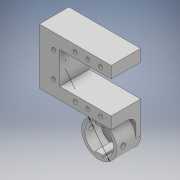
# Autodesk Inventor part: bottom
Saved by Autodesk Inventor 2018 (Build 220112000, 112)
## iProperties
Created: 2018-02-07
Part Number: bottom
Material: Générique
Document SubType Name: Modeling
Designer: Mephiro
Density: 1 g/cm^3
Appearance: Par défaut
Author: Mephiro
Autodesk Inventor part; units mm, degrees
ref_plane "YZ Plane" through (0, 0, 0) normal (1, 0, 0) x (0, 1, 0)
ref_plane "XZ Plane" through (0, 0, 0) normal (0, 1, 0) x (-1, 0, 0)
ref_plane "XY Plane" through (0, 0, 0) normal (0, 0, 1) x (1, 0, 0)
sketch "Esquisse1" plane through (0, 0, 0) normal (0, 1, 0) x (-1, 0, 0)
  circle A0 centre (0, 0) radius 11
  circle A1 centre (0, 0) radius 9.5
  dimension "d0" = 22
  dimension "d1" = 19
  constraints: 2 centre point, 2 coincident
  measures "d0" diameter of A0
  measures "d1" diameter of A1
extrude "Extrusion1" add sketch "Esquisse1" along normal blind 5 contours A0 | A1
sketch "Esquisse2" plane through (0, 0, 0) normal (0, -1, 0) x (1, 0, 0)
  circle A0 centre (0, 0) radius 11
  dimension "d5" = 22
  constraints: 1 centre point, 1 coincident
  measures "d5" diameter of A0
extrude "Extrusion2" add sketch "Esquisse2" along normal blind 10
sketch "Esquisse3" plane through (0, -10, 0) normal (0, -1, 0) x (1, 0, 0)
  arc A0 (2.4, -8.6741) -> (2.4, 8.6741) centre (0, 0) ccw
  arc A1 (-2.4, 8.6741) -> (-2.4, -8.6741) centre (0, 0) ccw
  line L0 (-2.4, -8.6741) -> (-2.4, -7.4241)
  line L1 (-2.4, -7.4241) -> (2.4, -7.4241)
  line L2 (2.4, -7.4241) -> (2.4, -8.6741)
  line L3 (-2.4, 8.6741) -> (-2.4, 7.4241)
  line L4 (-2.4, 7.4241) -> (2.4, 7.4241)
  line L5 (2.4, 7.4241) -> (2.4, 8.6741)
  dimension "d23" = 9
  dimension "d24" = 9
  dimension "d30" = 1.25
  dimension "d31" = 1.25
  dimension "d32" = 4.8
  dimension "d33" = 2.4
  dimension "d34" = 2.4
  dimension "d35" = 4.8
  constraints: 12 end point, 4 point on circle, 2 centre point, 2 parallel, 1 coincident
  measures "d23" radius of A0
  measures "d24" radius of A1
  measures "d30" distance of L1.end L2.end
  measures "d31" distance of L3.start L3.end
  measures "d32" distance of L2.end L0.start
  measures "d33" horizontal distance of L0.start point (0, 0)
  measures "d34" horizontal distance of point (0, 0) L3.start
  measures "d35" distance of L5.end L3.start
extrude "Extrusion3" cut sketch "Esquisse3" against normal blind 10
sketch "Esquisse5" plane through (0, 0, 0) normal (1, 0, 0) x (0, 1, 0)
  circle A0 centre (-6, 0) radius 1.5
  line L0 (0, -8.6741) -> (0, 8.6741) projected
  point P0 (0, 0)
  point P1 (0, -8.5184)
  point P2 (0, 8.5184)
  dimension "d26" = 3
  dimension "d27" = 6
  constraints: 1 centre point
  measures "d26" diameter of A0
  measures "d27" distance from line of L0 A0.centre
extrude "Extrusion5" cut sketch "Esquisse5" along normal mid plane 30
sketch "Esquisse14" plane through (41.6905, 5, 9.6899) normal (0, 1, 0) x (0, 0, -1)
  line L0 (-37.8101, 30.6905) -> (-2.8101, 30.6905)
  line L1 (-2.8101, 30.6905) -> (-2.8101, 75.6905)
  line L2 (-2.8101, 75.6905) -> (-37.8101, 75.6905)
  line L3 (-37.8101, 75.6905) -> (-37.8101, 30.6905)
  line L4 (-37.8101, 30.6905) -> (-37.8101, 75.6905)
  line L5 (-45, 30.6905) -> (-37.8101, 30.6905)
  circle A0 centre (9.6899, 41.6905) radius 11 projected
  point P0 (0, 0)
  dimension "d107" = 35
  dimension "d106" = 45
  dimension "d139" = 11
  dimension "d140" = 12.5
  constraints: 12 end point, 2 collinear, 2 parallel, 1 horizontal, 1 perpendicular
  measures "d107" distance of L0.start L0.end
  measures "d106" distance of L2.end L0.start
  measures "d139" distance from line of A0.centre L0
  measures "d140" distance from line of L1 A0.centre
extrude "Extrusion11" add sketch "Esquisse14" against normal blind 3 contours L3 L2 L1 L0
sketch "Esquisse18" plane through (0, 5, 12.5) normal (0, 0, -1) x (-1, 0, 0)
  line L0 (34, -3) -> (-11, -3) projected
  line L1 (11.3351, 0) -> (-11, 0)
  line L2 (-11, 0) -> (-11, -3)
  line L3 (-11, -3) -> (11.3351, -3)
  line L4 (11.3351, -3) -> (11.3351, 0)
  point P0 (0, -5)
  point P1 (0, -3)
  constraints: 8 end point, 2 parallel, 1 horizontal, 1 perpendicular
extrude "Extrusion14" add sketch "Esquisse18" along normal blind 12.5
sketch "Esquisse19" plane through (41.6905, 2, 9.6899) normal (0, -1, 0) x (1, 0, 0)
  line L0 (-30.6905, 28.8101) -> (-30.6905, 37.8101) projected
  line L1 (-75.6905, 2.8101) -> (-75.6905, 37.8101) projected
  line L2 (-30.6905, 37.8101) -> (-75.6905, 37.8101)
  line L3 (-75.6905, 37.8101) -> (-75.6905, 2.8101)
  line L4 (-75.6905, 2.8101) -> (-30.6905, 2.8101)
  line L5 (-30.6905, 2.8101) -> (-30.6905, 37.8101)
  point P0 (-41.6905, -9.6899)
  constraints: 8 end point, 2 parallel, 1 horizontal, 1 perpendicular
extrude "Extrusion15" add sketch "Esquisse19" along normal blind 15.5
sketch "Esquisse15" plane through (2.4261, 2, 9.0864) normal (0, -1, 0) x (0, 0, -1)
  line L0 (-20.9136, -42.6461) -> (-20.9136, -17.7284)
  line L1 (-34.4136, -42.6461) -> (-34.4136, 8.5739)
  line L2 (-7.4136, -42.6461) -> (-7.4136, 8.5739)
  line L3 (-47.9136, -27.4261) -> (-2.9136, -27.4261)
  line L4 (-37.9136, 2.0739) -> (-2.9136, 2.0739)
  line L5 (-20.9136, -17.7284) -> (-20.9136, 8.5739)
  circle A0 centre (-20.9136, 8.5739) radius 10
  line L6 (-34.4136, -5.9261) -> (-7.4136, -5.9261)
  line L7 (-34.4136, -13.9261) -> (-7.4136, -13.9261)
  line L8 (-3.4136, 8.5739) -> (-38.4136, 8.5739) projected
  line L9 (-3.4136, -36.4261) -> (-3.4136, 8.5739) projected
  point P0 (-7.4136, 2.0739)
  point P1 (-34.4136, 2.0739)
  point P2 (-7.4136, 2.0739)
  point P3 (-28.9136, -27.4261)
  point P4 (-12.9136, -27.4261)
  dimension "d120" = 13.5
  dimension "d119" = 13.5
  dimension "d118" = 20
  dimension "d116" = 8
  dimension "d115" = 8
  dimension "d114" = 8
  dimension "d113" = 8
  dimension "d117" = 6.5
  dimension "d112" = 13.5
  dimension "d155" = 4
  constraints: 16 end point, 10 point on line, 6 coincident, 2 horizontal, 2 perpendicular, 2 vertical, 1 centre point
  measures "d120" distance between parallel lines of L1 L0
  measures "d119" distance between parallel lines of L2 L0
  measures "d118" diameter of A0
  measures "d116" distance from line of point (-28.914, -27.426) L0
  measures "d115" distance from line of L0 point (-12.914, -27.426)
  measures "d114" distance between parallel lines of L4 L6
  measures "d113" distance between parallel lines of L6 L7
  measures "d117" distance from line of L8 point (-34.414, 2.074)
  measures "d112" distance from line of point (-28.914, -27.426) L7
  measures "d155" distance between parallel lines of L9 L2
hole "Perçage3" at (-25, 2, 38) at (-25, 2, 22) at (4.5, 2, 43.5) at (4.5, 2, 16.5) at (-3.5, 2, 43.5) at (-3.5, 2, 16.5) at (-11.5, 2, 43.5) at (-11.5, 2, 16.5) direction (0, 1, 0) diameter 2.5 end through all start extended yes
sketch "Esquisse17" plane through (41.6905, 2, 9.6899) normal (0, -1, 0) x (0, 0, -1)
  line L0 (-30.3101, -27.8905) -> (-10.3101, -27.8905)
  line L1 (-10.3101, -27.8905) -> (-10.3101, -62.8905)
  line L2 (-10.3101, -62.8905) -> (-30.3101, -62.8905)
  line L3 (-30.3101, -62.8905) -> (-30.3101, -27.8905)
  line L4 (-37.8101, -75.6905) -> (-2.8101, -75.6905) projected
  line L5 (-2.8101, -75.6905) -> (-2.8101, -23.6844) projected
  line L6 (-37.8101, -30.6905) -> (-37.8101, -75.6905) projected
  circle A0 centre (-28.3101, -66.6905) radius 1.25 projected
  point P0 (11.1035, -23.6844)
  point P1 (0.1035, -23.6844)
  dimension "d134" = 20
  dimension "d133" = 35
  dimension "d131" = 12.8
  dimension "d132" = 7.5
  dimension "d138" = 7.5
  dimension "d158" = 2.55
  constraints: 8 end point, 2 parallel, 1 horizontal, 1 perpendicular
  measures "d134" distance of L0.start L0.end
  measures "d133" distance of L2.end L0.start
  measures "d131" distance between parallel lines of L4 L2
  measures "d132" distance between parallel lines of L5 L1
  measures "d138" distance between parallel lines of L6 L3
  measures "d158" distance edge to line of A0 L2
extrude "Extrusion13" cut sketch "Esquisse17" against normal blind 10 and the other way blind 20 contours L0 L1 L2 L3
fillet "Congé1" radius 2 1 edges at (-11.3351, 3.5, 0)
fillet "Congé1" radius 5 1 edges at (-0.1676, 2, 12.5)
